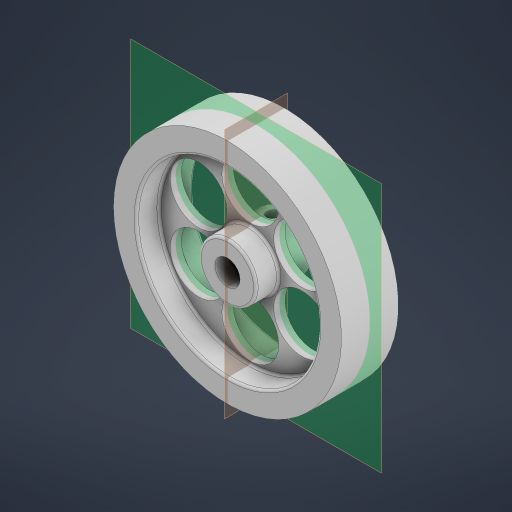
# Autodesk Inventor part: sf_Flywheel_1
Saved by Autodesk Inventor 2024 (Build 280153000, 153)
## iProperties
Created: 2024-03-20
Part Number: sf_Flywheel_1
Material: Generisch
Document SubType Name: Modeling
Designer: Simon
Density: 1 g/cm^3
Appearance: Vorgabe
Author: Simon
Autodesk Inventor part; units mm, degrees
ref_plane "XY Plane" through (0, 0, 0) normal (0, 0, 1) x (1, 0, 0)
sketch "Skizze1" plane through (0, 0, 0) normal (0, 1, 0) x (-1, 0, 0)
  circle A0 centre (0, 0) radius 50
  circle A1 centre (0, 0) radius 40
  circle A2 centre (0, 0) radius 12.5
  circle A3 centre (0, 0) radius 5.5
  dimension "d0" = 100
  dimension "d1" = 80
  dimension "d2" = 25
  dimension "d3" = 11
  constraints: 4 centre point, 4 coincident
  measures "d0" diameter of A0
  measures "d1" diameter of A1
  measures "d2" diameter of A2
  measures "d3" diameter of A3
extrude "Extrusion1" add sketch "Skizze1" along normal mid plane 25
sketch "Skizze2" plane through (0, 0, 0) normal (0, 1, 0) x (-1, 0, 0)
  circle A0 centre (0, 0) radius 40 projected
  circle A1 centre (0, 0) radius 12.5 projected
extrude "Extrusion2" add sketch "Skizze2" along normal mid plane 5
sketch "Skizze3" plane through (0, 0, 0) normal (0, 1, 0) x (-1, 0, 0)
  circle A0 centre (0, 0) radius 26.25 construction
  circle A1 centre (0, 26.25) radius 12.5
  circle A2 centre (0, 0) radius 26.25 construction
  circle A3 centre (-22.7332, 13.125) radius 12.5
  circle A4 centre (0, 0) radius 26.25 construction
  circle A5 centre (-22.7332, -13.125) radius 12.5
  circle A6 centre (0, 0) radius 26.25 construction
  circle A7 centre (0, -26.25) radius 12.5
  circle A8 centre (0, 0) radius 26.25 construction
  circle A9 centre (22.7332, -13.125) radius 12.5
  circle A10 centre (0, 0) radius 26.25 construction
  circle A11 centre (22.7332, 13.125) radius 12.5
  dimension "d8" = 52.5
  dimension "d9" = 25
  dimension "d12" = 360
  constraints: 6 centre point, 2 vertical alignment, 1 coincident, 41 other
  measures "d9" diameter of A1
extrude "Extrusion3" cut sketch "Skizze3" along normal mid plane 5
sketch "Skizze4" plane through (0, 0, 0) normal (1, 0, 0) x (0, 1, 0)
  line L0 (12.5, 5.5) -> (-12.5, 5.5) projected
  line L1 (4.5, 19.5) -> (9.5, 19.5) construction
  line L2 (9.5, 19.5) -> (9.5, 5.5) construction
  line L3 (9.5, 5.5) -> (4.5, 5.5) construction
  line L4 (4.5, 5.5) -> (4.5, 19.5) construction
  line L5 (2.5, 12.5) -> (12.5, 12.5) projected
  line L6 (9.5, 12.5) -> (5.4585, 5.5)
  line L7 (9.5, 12.5) -> (17.5829, 12.5) construction
  line L8 (5.4585, 5.5) -> (-0.0415, 5.5)
  line L9 (9.5, 12.5) -> (4.5, 12.5)
  line L10 (4.5, 12.5) -> (0.4585, 5.5)
  line L11 (4.5, 12.5) -> (12.5829, 12.5) construction
  line L12 (0.4585, 5.5) -> (5.4585, 5.5)
  line L13 (2.9585, 5.5) -> (7, 12.5) construction
  line L14 (7.4793, 9) -> (5.6043, 10.0825)
  line L15 (11.3125, 15.6393) -> (3.646, 2.3607)
  line L16 (3.646, 2.3607) -> (1.771, 3.4432)
  line L17 (1.771, 3.4432) -> (9.4375, 16.7219)
  line L18 (9.4375, 16.7219) -> (11.3125, 15.6393)
  line L19 (11.3125, 15.6393) -> (1.771, 3.4432) construction
  line L20 (3.646, 2.3607) -> (9.4375, 16.7219) construction
  point P0 (0, 0)
  point P1 (6.5418, 9.5413)
  dimension "d16" = 5
  dimension "d17" = 120
  dimension "d18" = 5.5
  dimension "d19" = 120
  constraints: 38 end point, 8 point on line, 7 midpoint, 5 parallel, 3 horizontal, 3 perpendicular, 2 collinear, 2 equal length
  measures "d16" distance of L2.end L3.end
  measures "d17" angle of L6 L7
  measures "d18" distance of L6.end L8.end
  measures "d19" angle of L10 L11
revolve "Umdrehung1" cut sketch "Skizze4" angle 360 about axis through (0, 1.771, 3.4432) along (0, 0.5, 0.8660254) contours L15 L16 L17 L0 | L0 L17 L14 L6 | L14 L17 L5 L6 | L5 L17 L18 L15
fillet "Rundung1" radius 1 8 edges at (40, 2.5, 0) (12.5, 2.5, 0) (40, 12.5, 0) (12.5, -2.5, 0) (40, -2.5, 0) (12.5, -12.5, 0) (40, -12.5, 0) (12.5, 12.5, 0)
